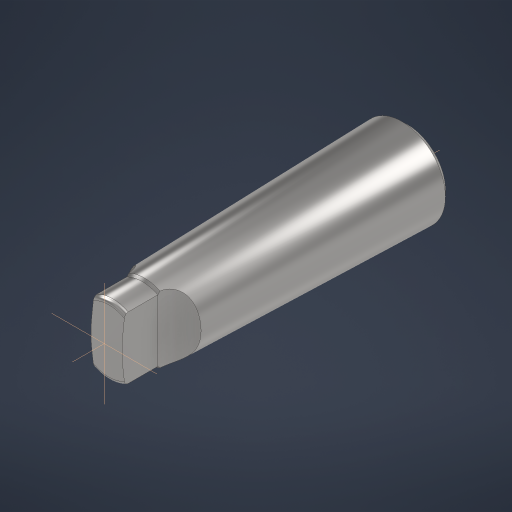
# Autodesk Inventor part: Part1
Saved by Autodesk Inventor 2023 (Build 270158000, 158)
## iProperties
Created: 2022-11-24
Part Number: Part1
Material: Steel, Alloy
Document SubType Name: Modeling
Designer: iusti
Density: 7.73 g/cm^3
Appearance: Semi-Polished
Author: iusti
Autodesk Inventor part; units mm, degrees
ref_plane "YZ Plane" through (0, 0, 0) normal (1, 0, 0) x (0, 1, 0)
ref_plane "XZ Plane" through (0, 0, 0) normal (0, 1, 0) x (-1, 0, 0)
ref_plane "XY Plane" through (0, 0, 0) normal (0, 0, 1) x (1, 0, 0)
sketch "Sketch1" plane through (0, 0, 0) normal (1, 0, 0) x (0, 1, 0)
  line L0 (0, 0) -> (18.2735, 0) construction
  line L1 (18.2735, 0) -> (18.8146, -20.5646) construction
  line L2 (22.3653, -155.5) -> (0, -155.5)
  line L3 (0, -155.5) -> (0, 0)
  line L4 (0, -186.6) -> (0, 31.1) projected
  line L5 (22.1995, -149.2) -> (0, -149.2) construction
  line L6 (-4.4731, 0) -> (26.8383, 0) construction
  line L7 (0, 0) -> (16.0387, -2.3398)
  line L8 (17.75, -4.3188) -> (17.75, -19.5)
  line L9 (17.75, -19.5) -> (18.8146, -20.5646)
  line L10 (18.8146, -20.5646) -> (22.3653, -155.5)
  arc A0 (17.75, -4.3188) -> (16.0387, -2.3398) centre (15.75, -4.3188) ccw
  dimension "d0" = 155.5
  dimension "d1" = 36.547
  dimension "d2" = 44.399
  dimension "d3" = 149.2
  dimension "d4" = 19.5
  dimension "d5" = 35.5
  dimension "d6" = 45
  dimension "d7" = 8.3
  dimension "d8" = 2
  constraints: 18 end point, 3 point on line, 2 collinear, 2 perpendicular, 2 point on circle, 2 tangent, 1 centre point, 1 horizontal, 1 parallel, 1 vertical
  measures "d0" distance of L2.end L0.start
  measures "d1" diameter of L0.end L3
  measures "d2" diameter of L5.start L3
  measures "d3" distance between parallel lines of L5 L0
  measures "d4" vertical distance of L0.end L8.end
  measures "d5" diameter of L8 L3
  measures "d6" angle of L9 L8
  measures "d7" angle of L7 L0
  measures "d8" radius of A0
revolve "Revolution1" add sketch "Sketch1" angle 360 about axis through (0, 0, -155.5) along (0, 0, 1)
chamfer "Chamfer1" distance 3 angle 45 1 edges at (0, -22.3653, -155.5)
sketch "Sketch3" plane through (0, 0, 0) normal (0, 1, 0) x (-1, 0, 0)
  line L0 (7.95, 0) -> (7.95, -19.5)
  arc A0 (7.95, -19.5) -> (19.5695, -30.4825) centre (18.95, -19.5) ccw
  line L1 (19.5695, -30.4825) -> (19.5695, 0)
  line L2 (19.5695, 0) -> (7.95, 0)
  line L3 (0, -186.6) -> (0, 31.1) projected
  line L4 (31.8888, 0) -> (-31.3156, 0) projected
  point P0 (0, 0)
  dimension "d19" = 15.9
  dimension "d20" = 30.5
  dimension "d21" = 11
  constraints: 6 end point, 2 point on circle, 2 vertical, 1 centre point, 1 collinear, 1 perpendicular, 1 tangent
  measures "d19" diameter of L0 L3
  measures "d21" radius of A0
extrude "Extrusion2" cut sketch "Sketch3" along normal through all both and the other way through all
mirror "Mirror2" about plane through (0, 0, 0) normal (1, 0, 0) of "Extrusion2"
body "Solid1"
